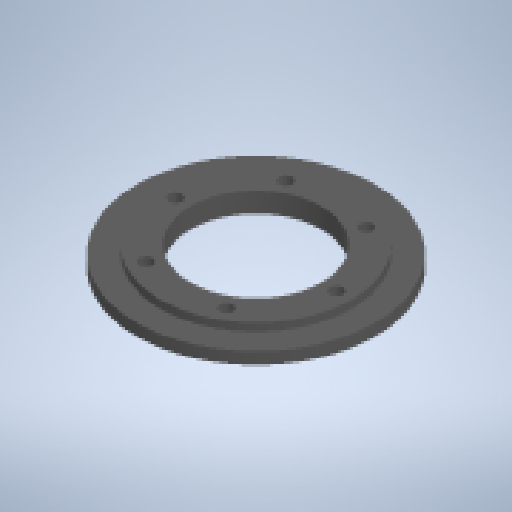
# Autodesk Inventor part: sholder_joint_c
Saved by Autodesk Inventor 2024.1 (Build 281209000, 209)
## iProperties
Created: 2024-02-14
Part Number: sholder_joint_c
Material: 一般
Document SubType Name: Sheet Metal
Designer: hibik
Density: 1 g/cm^3
Sheet Metal Rule: Default_mm
Appearance: 既定
Author: hibik
Autodesk Inventor part; units mm, degrees
ref_plane "YZ Plane" through (0, 0, 0) normal (1, 0, 0) x (0, 1, 0)
ref_plane "XZ Plane" through (0, 0, 0) normal (0, 1, 0) x (-1, 0, 0)
ref_plane "XY Plane" through (0, 0, 0) normal (0, 0, 1) x (1, 0, 0)
sketch "スケッチ1" plane through (0, 0, 0) normal (0, 1, 0) x (-1, 0, 0)
  circle A0 centre (0, 0) radius 8.25
  circle A1 centre (0, 0) radius 15
  circle A2 centre (0, 0) radius 12
  dimension "d0" = 16.5
  dimension "d1" = 30
  dimension "d5" = 24
  constraints: 6 coincident, 3 centre point
  measures "d0" diameter of A0
  measures "d1" diameter of A1
  measures "d5" diameter of A2
extrude "押し出し1" add sketch "スケッチ1" along normal blind 1.5 contours A1 | A2
extrude "押し出し2" add sketch "スケッチ1" along normal blind 2.5 contours A2
sketch "スケッチ2" plane through (0, 0, 0) normal (0, -1, 0) x (1, 0, 0)
  circle A0 centre (5.0625, -8.7685) radius 1 construction
  circle A1 centre (10.125, 0) radius 1 construction
  circle A2 centre (5.0625, 8.7685) radius 1 construction
  circle A3 centre (-5.0625, 8.7685) radius 1 construction
  circle A4 centre (-10.125, 0) radius 1 construction
  circle A5 centre (-5.0625, -8.7685) radius 1 construction
  circle A6 centre (10.125, 0) radius 0.8
  circle A7 centre (5.0625, -8.7685) radius 0.8
  circle A8 centre (-5.0625, -8.7685) radius 0.8
  circle A9 centre (-10.125, 0) radius 0.8
  circle A10 centre (-5.0625, 8.7685) radius 0.8
  circle A11 centre (5.0625, 8.7685) radius 0.8
  point P0 (0, 0)
  dimension "d10" = 1.6
  dimension "d11" = 1.6
  dimension "d12" = 1.6
  dimension "d13" = 1.6
  dimension "d14" = 1.6
  dimension "d15" = 1.6
  constraints: 6 centre point, 6 coincident
  measures "d10" diameter of A6
  measures "d11" diameter of A7
  measures "d12" diameter of A8
  measures "d13" diameter of A9
  measures "d14" diameter of A10
  measures "d15" diameter of A11
extrude "押し出し3" cut sketch "スケッチ2" against normal through all
equation "\"BendRadius\" = Thickness"
equation "\"BendReliefWidth\" = Thickness"
equation "\"BendReliefDepth\" = 0.5 * Thickness"
equation "\"CornerReliefSize\" = 4 * Thickness"
equation "\"MinimumRemnant\" = 2 * Thickness"
equation "\"TransitionRadius\" = BendRadius"
equation "\"JacobiRadiusSize\" = BendRadius"
equation "\"GapSize\" = Thickness"
equation "\"Thickness\" = 1.5"
